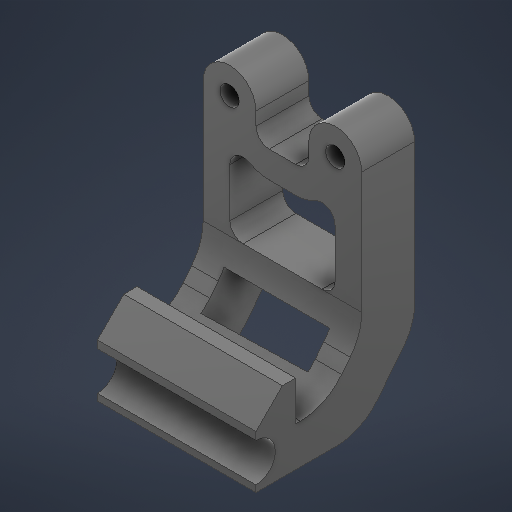
# Autodesk Inventor part: Rear Jaw
Saved by Autodesk Inventor 2025 (Build 290162000, 162)
## iProperties
Created: 2025-01-03
Part Number: Rear Jaw
Material: Generic
Document SubType Name: Modeling
Designer: Juan
Density: 1 g/cm^3
Appearance: Default
Author: Juan
Autodesk Inventor part; units mm, degrees
ref_plane "YZ Plane" through (0, 0, 0) normal (1, 0, 0) x (0, 1, 0)
ref_plane "XZ Plane" through (0, 0, 0) normal (0, 1, 0) x (-1, 0, 0)
ref_plane "XY Plane" through (0, 0, 0) normal (0, 0, 1) x (1, 0, 0)
sketch "Sketch1" plane through (0, 0, 0) normal (0, 0, 1) x (1, 0, 0)
  line L0 (0, 0) -> (12.7, 0)
  line L1 (0, 0) -> (-12.7, 0)
  circle A0 centre (-12.7, 0) radius 2.3241
  circle A1 centre (12.7, 0) radius 2.3241
  line L2 (-12.7, 0) -> (-6.35, 0)
  circle A2 centre (-12.7, 0) radius 6.35
  circle A3 centre (12.7, 0) radius 6.35
  line L3 (-12.7, -6.35) -> (-10.8231, -6.35)
  line L4 (-10.8231, -6.35) -> (12.7, -6.35)
  line L5 (-19.05, 0) -> (19.05, 0)
  line L6 (19.05, 0) -> (19.05, -50.8)
  line L7 (19.05, -50.8) -> (-19.05, -50.8)
  line L8 (-19.05, -50.8) -> (-19.05, 0)
  line L9 (-6.35, 0) -> (-6.35, -6.35)
  line L10 (6.35, 0) -> (6.35, -6.35)
  dimension "d0" = 12.7
  dimension "d1" = 12.7
  dimension "d2" = 4.6482
  dimension "d3" = 4.6482
  dimension "d5" = 12.7
  dimension "d6" = 50.8
  constraints: 22 end point, 5 point on circle, 4 centre point, 4 coincident, 4 point on line, 3 horizontal, 3 perpendicular, 3 tangent, 2 parallel, 1 midpoint
  measures "d0" distance of L0.start L0.end
  measures "d1" distance of L0.start L1.end
  measures "d2" diameter of A0
  measures "d3" diameter of A1
  measures "d5" diameter of A3
  measures "d6" distance of L5.end L6.end
extrude "Extrusion1" add sketch "Sketch1" along normal blind 12.7 contours A3 L5 A1 L0 | L0 A1 L5 A3 | A3 L4 L10 | A2 L5 A0 L1 | L1 A0 L5 A2 | L9 L4 L3 A2 | L6 L7 L8 A2 L3 L4 A3
fillet "Fillet1" radius 3.175 2 edges at (6.35, -6.35, 6.35) (-6.35, -6.35, 6.35)
sketch "Sketch2" plane through (-19.05, -50.8, 0) normal (-1, 0, 0) x (0, 0, 1)
  line L0 (12.7, 50.8) -> (12.7, 0) projected
  line L1 (0, 0) -> (12.7, 0) projected
  line L2 (12.7, 0) -> (38.1, 0)
  line L3 (38.1, 0) -> (38.1, 6.35)
  line L4 (38.1, 6.35) -> (12.7, 6.35)
  point P0 (0, 50.8)
  dimension "d10" = 25.4
  dimension "d11" = 6.35
  constraints: 6 end point, 1 horizontal, 1 perpendicular, 1 point on line, 1 vertical
  measures "d10" distance of L0.end L2.end
  measures "d11" distance of L2.end L3.end
extrude "Extrusion2" add sketch "Sketch2" against normal up to surface (38.1 mm away)
sketch "Sketch3" plane through (-19.05, -44.45, 38.1) normal (0, 1, 0) x (1, 0, 0)
  line L0 (38.1, 0) -> (38.1, 25.4) projected
  line L1 (0, 25.4) -> (38.1, 25.4) projected
  line L2 (0, 0) -> (0, 25.4) projected
  line L3 (0, 0) -> (38.1, 0) projected
  line L4 (38.1, 0) -> (0, 0)
  line L5 (0, 0) -> (0, 9.525)
  line L6 (0, 9.525) -> (38.1, 9.525)
  line L7 (38.1, 9.525) -> (38.1, 0)
  point P0 (19.05, 38.1)
  dimension "d14" = 9.525
  constraints: 8 end point, 2 parallel, 1 horizontal, 1 perpendicular, 1 point on line
  measures "d14" distance of L2.start L5.end
extrude "Extrusion3" add sketch "Sketch3" along normal blind 9.525 contours L3 L2 L6 L0
sketch "Sketch4" plane through (-19.05, -50.8, 0) normal (0, -1, 0) x (1, 0, 0)
  line L0 (0, 0) -> (38.1, 0) projected
  line L1 (38.1, 0) -> (38.1, 38.1) projected
  line L2 (0, 38.1) -> (38.1, 38.1) projected
  line L3 (0, 0) -> (0, 38.1) projected
  point P0 (19.05, 0)
extrude "Extrusion4" add sketch "Sketch4" along normal blind 3.175
chamfer "Chamfer1" distance 6.35 angle 45 1 edges at (0, -34.925, 38.1)
sketch "Sketch5" plane through (-19.05, 0, 0) normal (-1, 0, 0) x (0, 0, 1)
  line L0 (38.1, -53.975) -> (0, -53.975) projected
  line L1 (38.1, -53.975) -> (38.1, -52.3875)
  line L2 (38.1, -53.975) -> (38.1, -41.275) projected
  line L3 (38.1, -52.3875) -> (38.1, -47.7393)
  circle A0 centre (38.1, -47.7393) radius 4.6482
  point P0 (0, 0)
  point P1 (38.1, -43.0911)
  dimension "d22" = 1.5875
  dimension "d23" = 4.6482
  constraints: 4 end point, 2 point on line, 1 coincident, 3 other
  measures "d22" distance of L0.start L1.end
  measures "d23" distance of L1.end L3.end
extrude "Extrusion5" cut sketch "Sketch5" against normal through all contours A0 L2 picked at (35.7974, -45.6994)
sketch "Sketch6" plane through (-19.05, 0, 0) normal (-1, 0, 0) x (0, 0, 1)
  arc A0 (38.1, -43.0911) -> (38.1, -52.3875) centre (38.1, -47.7393) ccw projected
  line L0 (38.1, -43.0911) -> (38.1, -41.275) projected
  line L1 (31.75, -34.925) -> (38.1, -41.275) projected
  line L2 (28.575, -34.925) -> (31.75, -34.925) projected
  line L3 (28.575, -44.45) -> (28.575, -34.925) projected
  line L4 (28.575, -44.45) -> (12.7, -44.45) projected
  line L5 (12.7, 0) -> (12.7, -44.45) projected
  line L6 (0, 0) -> (12.7, 0) projected
  line L7 (0, 0) -> (0, -53.975) projected
  line L8 (38.1, -53.975) -> (0, -53.975) projected
  line L9 (38.1, -53.975) -> (38.1, -52.3875) projected
  line L10 (12.7, -53.975) -> (0, -38.1)
  line L11 (22.617, -46.0414) -> (9.917, -30.1664)
  point P0 (0, 0)
  point P1 (21.3439, -44.45)
  point P2 (12.7, -33.6451)
  dimension "d26" = 12.7
  constraints: 4 end point, 3 point on line, 1 parallel
  measures "d26" distance between parallel lines of L10 L11
extrude "Extrusion6" cut sketch "Sketch6" against normal through all contours L8 L7 L10
extrude "Extrusion7" add sketch "Sketch6" against normal up to surface (38.1 mm away) contours L4 L5 L11
fillet "Fillet2" radius 12.7 4 edges at (0, -38.1, 0) (0, -53.975, 12.7) (0, -33.6451, 12.7) (0, -44.45, 21.3439)
sketch "Sketch7" plane through (0, 0, 12.7) normal (0, 0, 1) x (1, 0, 0)
  line L0 (19.05, -29.1902) -> (-19.05, -29.1902) projected
  line L1 (19.05, -29.1902) -> (19.05, 0) projected
  arc A0 (19.05, 0) -> (6.35, 0) centre (12.7, 0) ccw projected
  line L2 (6.35, 0) -> (6.35, -3.175) projected
  arc A1 (3.175, -6.35) -> (6.35, -3.175) centre (3.175, -3.175) ccw projected
  line L3 (3.175, -6.35) -> (-3.175, -6.35) projected
  arc A2 (-6.35, -3.175) -> (-3.175, -6.35) centre (-3.175, -3.175) ccw projected
  line L4 (-6.35, -3.175) -> (-6.35, 0) projected
  arc A3 (-6.35, 0) -> (-19.05, 0) centre (-12.7, 0) ccw projected
  line L5 (-19.05, 0) -> (-19.05, -29.1902) projected
  circle A4 centre (-12.7, 0) radius 2.3241 projected
  circle A5 centre (12.7, 0) radius 2.3241 projected
  line L6 (-3.175, -12.7649) -> (3.175, -12.7649)
  arc A6 (3.175, -12.7649) -> (12.6351, -4.7474) centre (3.175, -3.175) ccw
  line L7 (12.6351, -4.7474) -> (12.6351, -22.7753)
  line L8 (12.6351, -22.7753) -> (-12.6351, -22.7753)
  line L9 (-12.6351, -22.7753) -> (-12.6351, -4.7474)
  arc A7 (-12.6351, -4.7474) -> (-3.175, -12.7649) centre (-3.175, -3.175) ccw
  line L10 (-12.6351, -22.7753) -> (-12.6351, -29.1902)
  line L11 (12.6351, -29.1902) -> (12.6351, -22.7753)
  line L12 (12.6351, -29.1902) -> (-12.6351, -29.1902)
  point P0 (0, 0)
  constraints: 14 end point, 4 point on circle, 3 perpendicular, 2 centre point, 2 point on line, 5 other
extrude "Extrusion8" cut sketch "Sketch7" against normal through all contours L0 L10 L8 L11 | L8 L9 A7 L6 A6 L7
fillet "Fillet3" radius 3.175 2 edges at (-12.6351, -4.7474, 6.35) (12.6351, -4.7474, 6.35)
fillet "Fillet4" radius 3.175 2 edges at (12.6351, -29.1902, 6.35) (-12.6351, -29.1902, 6.35)
sketch "Sketch8" plane through (-19.05, -34.925, 31.75) normal (0, 0.7071, 0.7071) x (1, 0, 0)
  ellipse E0 centre (31.75, 38.1661) end of major axis (29.4259, 38.1661) minor radius 1.6434 projected
  ellipse E1 centre (6.35, 38.1661) end of major axis (4.0259, 38.1661) minor radius 1.6434 projected
  line L0 (6.4149, 19.7706) -> (6.4149, 28.0648) projected
  ellipse E2 centre (9.5899, 28.0648) end of major axis (6.4149, 28.0648) minor radius 2.2451 (11.1532, 30.0189) -> (6.4149, 28.0648) ccw projected
  ellipse E3 centre (15.875, 35.921) end of major axis (25.4649, 35.921) minor radius 6.7811 (11.1532, 30.0189) -> (15.875, 29.1399) ccw projected
  line L1 (15.875, 29.1399) -> (22.225, 29.1399) projected
  ellipse E4 centre (22.225, 35.921) end of major axis (12.6351, 35.921) minor radius 6.7811 (22.225, 29.1399) -> (26.9468, 30.0189) ccw projected
  ellipse E5 centre (28.5101, 28.0648) end of major axis (25.3351, 28.0648) minor radius 2.2451 (31.6851, 28.0648) -> (26.9468, 30.0189) ccw projected
  line L2 (31.6851, 28.0648) -> (31.6851, 19.7706) projected
  ellipse E6 centre (28.5101, 19.7706) end of major axis (31.6851, 19.7706) minor radius 2.2451 (28.5101, 17.5255) -> (31.6851, 19.7706) ccw projected
  line L3 (38.1, 17.5255) -> (28.5101, 17.5255) projected
  line L4 (38.1, 17.5255) -> (38.1, 38.1661) projected
  ellipse E7 centre (31.75, 38.1661) end of major axis (38.1, 38.1661) minor radius 4.4901 (38.1, 38.1661) -> (25.4, 38.1661) ccw projected
  line L5 (25.4, 38.1661) -> (25.4, 35.921) projected
  ellipse E8 centre (22.225, 35.921) end of major axis (25.4, 35.921) minor radius 2.2451 (22.225, 33.676) -> (25.4, 35.921) ccw projected
  line L6 (22.225, 33.676) -> (15.875, 33.676) projected
  ellipse E9 centre (15.875, 35.921) end of major axis (19.05, 35.921) minor radius 2.2451 (12.7, 35.921) -> (15.875, 33.676) ccw projected
  line L7 (12.7, 35.921) -> (12.7, 38.1661) projected
  ellipse E10 centre (6.35, 38.1661) end of major axis (12.7, 38.1661) minor radius 4.4901 (12.7, 38.1661) -> (0, 38.1661) ccw projected
  line L8 (0, 38.1661) -> (0, 17.5255) projected
  line L9 (9.5899, 17.5255) -> (0, 17.5255) projected
  ellipse E11 centre (9.5899, 19.7706) end of major axis (12.7649, 19.7706) minor radius 2.2451 (6.4149, 19.7706) -> (9.5899, 17.5255) ccw projected
  line L10 (6.4149, 17.5255) -> (6.4149, 3.7029)
  line L11 (6.4149, 3.7029) -> (31.75, 4.1664)
  line L12 (31.75, 4.1664) -> (31.75, 17.5255)
  line L13 (6.4149, 17.5255) -> (31.75, 17.5255)
  line L14 (6.4149, 17.5255) -> (6.4149, 12.4851)
  line L15 (6.4149, 12.4851) -> (31.75, 12.4851)
  point P0 (19.05, 47.1463)
  constraints: 12 end point, 4 perpendicular, 4 point on line, 12 other
extrude "Extrusion9" cut sketch "Sketch8" against normal through all contours L15 L12 L11 L10
body "Solid1"
